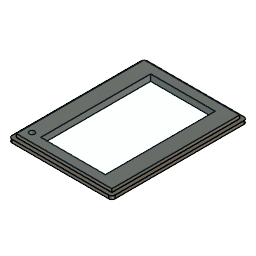
cover (Autodesk Fusion 360 design; units mm, degrees)
part number: 2026-04-23-02-04-09-797
Autodesk Fusion 360 part; units mm, degrees
sketch "草图1" plane through (0, 0, 0) normal (0, 0, 1) x (1, 0, 0)
  line L0 (0, 80) -> (160, 80)
  line L1 (160, 80) -> (160, -130)
  line L2 (160, -130) -> (0, -130)
  line L3 (0, -130) -> (0, 80)
  constraint horizontal L0
  constraint vertical L1
  constraint horizontal L2
  constraint vertical L3
extrude "拉伸1" add sketch "草图1" along normal blind 5
sketch "草图2" plane through (0, 0, 5) normal (0, 0, 1) x (-1, 0, 0)
  line L0 (0, 130) -> (-160, 130)
  line L1 (-160, 130) -> (-160, -80)
  line L2 (-160, -80) -> (0, -80)
  line L3 (0, -80) -> (0, 130)
  line L4 (-30, -60) -> (-130, -60)
  line L5 (-130, -60) -> (-130, 110)
  line L6 (-130, 110) -> (-30, 110)
  line L7 (-30, 110) -> (-30, -60)
  line L8 (-6, -74) -> (-154, -74)
  line L9 (-154, -74) -> (-154, 124)
  line L10 (-154, 124) -> (-6, 124)
  line L11 (-6, 124) -> (-6, -74)
  dimension "d3" = 148
  dimension "d4" = 198
  constraint horizontal L4
  constraint vertical L5
  constraint horizontal L6
  constraint vertical L7
  constraint horizontal L8
  constraint vertical L9
  constraint horizontal L10
  constraint vertical L11
  measures "d3" distance of L8.start L8.end
  measures "d4" distance of L8.start L10.end
extrude "拉伸2" add sketch "草图2" along normal blind 5 contours L8 L9 L10 L11
extrude "拉伸3" cut 1 faces at (63.3333, 3.3333, 5) along direction (0, 0, -1) blind 20
hole "孔1" at (16.7934, -110.3616, 10) direction (0, 0, -1) diameter 8 depth 20 tip angle 118
fillet "圆角1" radius 5 4 edges at (0, -130, 2.5) (0, 80, 2.5) (160, -130, 2.5) (160, 80, 2.5)
sketch "草图3" plane through (0, 0, 0) normal (0, 0, -1) x (1, 0, 0)
  arc A0 (155, -80) -> (160, -75) centre (155, -75) ccw
  line L0 (160, -75) -> (160, 125)
  arc A1 (160, 125) -> (155, 130) centre (155, 125) ccw
  line L1 (155, 130) -> (5, 130)
  arc A2 (5, 130) -> (0, 125) centre (5, 125) ccw
  line L2 (0, 125) -> (0, -75)
  arc A3 (0, -75) -> (5, -80) centre (5, -75) ccw
  line L3 (5, -80) -> (155, -80)
  circle A4 centre (16.7934, 110.3616) radius 4
  line L4 (130, -60) -> (30, -60)
  line L5 (30, -60) -> (30, 110)
  line L6 (30, 110) -> (130, 110)
  line L7 (130, 110) -> (130, -60)
  line L8 (129.8959, -63.2606) -> (30, -63.2606) construction
  line L9 (30, -63.2606) -> (30, -76.84) construction
  line L10 (30, -76.84) -> (129.8959, -76.84) construction
  line L11 (129.8959, -76.84) -> (129.8959, -63.2606) construction
  dimension "d14" = 6
  text T0 "Intelligent PM Detector" font "Arial" height 6 align centre middle in box 99.8959 x 13.5794 at (129.8959, -63.2606) x (-1, 0) y (0, -1) spacing 1
extrude "拉伸4" cut sketch "草图3" against normal blind 1.2 text T0
sketch "草图4" plane through (0, 0, 10) normal (0, 0, 1) x (-1, 0, 0)
  circle A0 centre (-16.7934, 110.3616) radius 4
  line L0 (-130, 110) -> (-30, 110)
  line L1 (-30, 110) -> (-30, -60)
  line L2 (-30, -60) -> (-130, -60)
  line L3 (-130, -60) -> (-130, 110)
  line L4 (-6, 124) -> (-154, 124)
  line L5 (-154, 124) -> (-154, -74)
  line L6 (-154, -74) -> (-6, -74)
  line L7 (-6, -74) -> (-6, 124)
equation "d15 = 'Intelligent PM Detector'"
